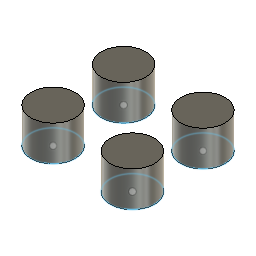
Case bottom (Autodesk Fusion 360 archive; units mm, degrees)
design "cyclinders"
part number: 2026-02-26-00-14-27-917
Autodesk Fusion 360 part; units mm, degrees
sketch "Sketch1" plane through (0, 0, 0) normal (0, 0, 1) x (1, 0, 0)
  circle A0 centre (6, 5) radius 2.5
  circle A1 centre (15, 5) radius 2.5
  circle A2 centre (6, 13) radius 2.5
  circle A3 centre (15, 13) radius 2.5
  dimension "d1" = 5
  dimension "d2" = 5
  dimension "d3" = 5
  dimension "d4" = 5
  measures "d1" diameter of A0
  measures "d2" diameter of A1
  measures "d3" diameter of A2
  measures "d4" diameter of A3
extrude "Extrude1" add sketch "Sketch1" along normal blind 4 contours A2 makes body 1
extrude "Extrude2" add sketch "Sketch1" along normal blind 4 separate body contours A0 makes body 2
extrude "Extrude3" add sketch "Sketch1" along normal blind 4 separate body contours A3 makes body 3
extrude "Extrude4" add sketch "Sketch1" along normal blind 4 separate body contours A1 makes body 4
